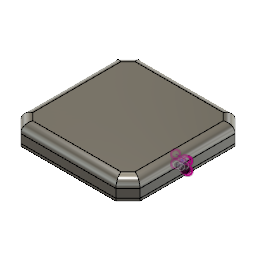
LightSwitch (Autodesk Fusion 360 design; units mm, degrees)
Autodesk Fusion 360 part; units mm, degrees
sketch "Sketch1" plane through (0, 0, 0) normal (0, 1, 0) x (1, 0, 0)
  line L0 (35, 35) -> (-35, -35) construction
  line L1 (-35, 35) -> (35, -35) construction
  line L2 (27.9289, -35) -> (35, -27.9289)
  line L3 (35, 27.9289) -> (27.9289, 35)
  line L4 (-27.9289, 35) -> (-35, 27.9289)
  line L5 (-35, -27.9289) -> (-27.9289, -35)
  line L6 (-35, 35) -> (-35, 27.9289)
  line L7 (-35, -27.9289) -> (-35, -35)
  line L8 (-35, 27.9289) -> (-35, -27.9289)
  line L9 (35, 35) -> (27.9289, 35)
  line L10 (-27.9289, 35) -> (-35, 35)
  line L11 (27.9289, 35) -> (-27.9289, 35)
  line L12 (-35, -35) -> (-27.9289, -35)
  line L13 (27.9289, -35) -> (35, -35)
  line L14 (-27.9289, -35) -> (27.9289, -35)
  line L15 (35, -35) -> (35, -27.9289)
  line L16 (35, 27.9289) -> (35, 35)
  line L17 (35, -27.9289) -> (35, 27.9289)
  line L18 (27.2919, 33.462) -> (-27.2919, 33.462)
  line L19 (-27.2919, 33.462) -> (-33.462, 27.2919)
  line L20 (-33.462, 27.2919) -> (-33.462, -27.2919)
  line L21 (-33.462, -27.2919) -> (-27.2919, -33.462)
  line L22 (-27.2919, -33.462) -> (27.2919, -33.462)
  line L23 (27.2919, -33.462) -> (33.462, -27.2919)
  line L24 (33.462, -27.2919) -> (33.462, 27.2919)
  line L25 (33.462, 27.2919) -> (27.2919, 33.462)
  dimension "d1" = 70
  dimension "d2" = 70
  dimension "d3" = 10
  dimension "d6" = 360
  dimension "d7" = 70
  dimension "d10" = 7.0711
  dimension "d11" = 1.538
extrude "Extrude1" add sketch "Sketch1" along normal blind 1.5 contours L2 L3 L4 L5 L8 L11 L14 L17 | L18 L19 L20 L21 L22 L23 L24 L25 makes body 1
extrude "Extrude2" add 1 faces at (-6.9526, 1.5, 9.3096) along direction (0, 1, 0) blind 10 on bodies 1 bodies 1
fillet "Fillet1" radius 5 8 edges at (0, 11.5, 35) (-31.4645, 11.5, 31.4645) (-35, 11.5, 0) (-31.4645, 11.5, -31.4645) (0, 11.5, -35) (31.4645, 11.5, 31.4645) (35, 11.5, 0) (31.4645, 11.5, -31.4645) on bodies 1
shell "Shell1" thickness 1.5 removed faces 0 bodies 1
ref_plane "WorkPlane1" through (31.4645, 1.5, -31.4645) normal (0, 1, 0) x (1, 0, 0)
split "Split1" by plane through (31.4645, 1.5, -31.4645) normal (0, 1, 0) bodies 1 makes body 2 at (10, 10, 8.6193)
sketch "Sketch3" plane through (0, 0, 0) normal (0, 0, 1) x (1, 0, 0)
  line L0 (33.5, 1.5) -> (33.5, 6.5)
  line L1 (35, 6.5) -> (27.9289, 6.5)
  line L2 (33.5, 1.5) -> (33.5, 3.5)
  line L3 (33.5, 3.5) -> (32.5, 3)
  line L4 (35, 1.5) -> (27.9289, 1.5)
  line L5 (33.5, 1.5) -> (32.4, 1.5)
  line L6 (31.9, 2) -> (31.9, 3.4501)
  line L7 (31.9, 3.4501) -> (31.9, 4)
  line L8 (31.9, 4) -> (33, 4)
  line L9 (33, 4) -> (31.9, 3.4501)
  line L10 (32.5, 2.5) -> (32.5, 3)
  line L11 (33.5, 1.5) -> (31, 1.5)
  line L12 (31, 4) -> (31, 2)
  arc A0 (31.9, 2) -> (32.4, 1.5) centre (32.4, 2) ccw
  line L13 (30.5, 1.5) -> (28.9, 1.5)
  arc A1 (30.5, 1.5) -> (31, 2) centre (30.5, 2) ccw
  line L14 (32.5, 2.5) -> (33.5, 1.7)
  line L15 (33, 4) -> (33, 4.5)
  line L16 (33, 4.5) -> (32, 5.5)
  line L17 (32, 5.5) -> (31.5, 5.5)
  line L18 (31.5, 5.5) -> (31, 4.5)
  line L19 (31, 4.5) -> (31, 4)
  dimension "d20" = 0.5
  dimension "d21" = 0.5
  measures "d20" radius of A0
  measures "d21" radius of A1
extrude "Extrude3" add sketch "Sketch3" along normal mid plane 50 contours L4 L6 L7 L8 L11 L12 A0 A1 L15 L16 L17 L18 L19 | L7 L8 L9 bodies 1
extrude "Extrude4" add sketch "Sketch3" along normal mid plane 50 contours L0 L2 L3 L10 L14 bodies 2
extrude "Extrude6" cut sketch "Sketch3" along normal mid plane 15 bodies 2 1
pattern_circular "C-Pattern1" count 4 over 360 about axis through (0, 1.75, 0) along (0, 1, 0) of "Extrude3", "Extrude4", "Extrude6"
sketch "Sketch5" plane through (0, 0, 0) normal (0, 1, 0) x (1, 0, 0)
  line L0 (27.9289, 35) -> (-27.9289, 35)
  line L1 (-7.6716, 35) -> (8, 35)
  line L2 (0, 35) -> (0, 30)
  line L3 (3.75, 31.5) -> (-3.75, 31.5)
  line L4 (-5, 30.25) -> (-5, 29.75)
  line L5 (-3.75, 28.5) -> (3.75, 28.5)
  line L6 (5, 29.75) -> (5, 30.25)
  line L7 (5, 31.5) -> (-5, 28.5) construction
  line L8 (-5, 31.5) -> (5, 28.5) construction
  arc A0 (5, 30.25) -> (3.75, 31.5) centre (3.75, 30.25) ccw
  arc A1 (3.75, 28.5) -> (5, 29.75) centre (3.75, 29.75) ccw
  arc A2 (-5, 29.75) -> (-3.75, 28.5) centre (-3.75, 29.75) ccw
  arc A3 (-3.75, 31.5) -> (-5, 30.25) centre (-3.75, 30.25) ccw
  line L9 (0, 0) -> (9, 0)
  line L10 (-3.75, -28.5) -> (3.75, -28.5)
  arc A4 (-5, -30.25) -> (-3.75, -31.5) centre (-3.75, -30.25) ccw
  line L11 (-5, -30.25) -> (-5, -29.75)
  arc A5 (-3.75, -28.5) -> (-5, -29.75) centre (-3.75, -29.75) ccw
  line L12 (0, -35) -> (0, -30)
  line L13 (3.75, -31.5) -> (-3.75, -31.5)
  line L14 (5, -29.75) -> (5, -30.25)
  line L15 (-5, -31.5) -> (5, -28.5) construction
  arc A6 (3.75, -31.5) -> (5, -30.25) centre (3.75, -30.25) ccw
  arc A7 (5, -29.75) -> (3.75, -28.5) centre (3.75, -29.75) ccw
  line L16 (5, -31.5) -> (-5, -28.5) construction
  line L17 (35, -27.9289) -> (35, 27.9289)
  line L18 (35, -27.9289) -> (35, 27.9289)
  line L19 (35, 0) -> (27.9289, 0)
  line L20 (35, -7.15) -> (35, 7)
  line L21 (35, 0) -> (25, 0)
  circle A8 centre (25, 0) radius 1.5
  line L22 (0, 0) -> (0, 8)
  circle A9 centre (-25, 0) radius 1.5
  point P0 (-20, 0)
  point P1 (-20, 0)
  dimension "d33" = 10
  dimension "d34" = 3
  dimension "d35" = 1.25
  dimension "d36" = 5
  dimension "d37" = 3
  dimension "d38" = 10
  dimension "d39" = 3
  measures "d35" radius of A0
  measures "d37" distance of L3 L5
  measures "d39" diameter of A8
extrude "Extrude7" cut sketch "Sketch5" along normal blind 10 bodies 1
